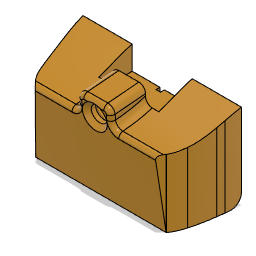
Nase+_ohne_Cam (Autodesk Fusion 360 design; units mm, degrees)
Autodesk Fusion 360 part; units mm, degrees
sketch "Skizze1" plane through (0, 0, 0) normal (1, 0, 0) x (0, 0, -1)
  line L0 (-230.1322, -57.5923) -> (-230.1322, 8.8027)
  spline S0 degree 3 poles (-230.1322, -57.5923) (-230.1323, -58.3551) (-230.2195, -59.1172) (-230.681, -61.096) (-231.1997, -62.2622) (-232.679, -64.3902) (-233.6453, -65.3172) (-235.732, -66.6453) (-236.7991, -67.0899) (-238.6452, -67.5093) (-239.3882, -67.5923) (-240.1323, -67.5923) knots -3.547857 -3.547857 -3.547857 -3.547857 -3.317948 -3.317948 -2.938178 -2.938178 -2.539541 -2.539541 -2.193953 -2.193953 -1.968953 -1.968953 -1.968953 -1.968953
  line L1 (-285.1866, -67.5923) -> (-240.1323, -67.5923)
  line L2 (-285.1866, -67.5923) -> (-291.9232, 9.4077)
  line L3 (-291.9232, 9.4077) -> (-255.1322, 12.6265)
  line L4 (-255.1322, 12.6265) -> (-255.1322, -10.5402)
  line L5 (-255.1322, -10.5402) -> (-230.1322, -10.5402)
  line L6 (-235.8283, -10.5402) -> (-205.3183, -10.5402)
  dimension "d33" = 95
  dimension "d34" = 77
  dimension "d35" = 25
  constraint coincident L1.start L2.start
  constraint perpendicular L2 L3
  constraint coincident L0 L5.end
  constraint perpendicular L0 L5
  constraint vertical L4
  constraint collinear L5 L6
  measures "d33" angle of L1 L2
  measures "d34" vertical distance of L1.start L2.end
  measures "d35" distance of L4.end L5.end
extrude "Extrusion1" add sketch "Skizze1" along normal blind 75
sketch "Skizze2" plane through (75, 0, 0) normal (1, 0, 0) x (0, 0, -1)
  line L0 (-285.1866, -67.5923) -> (-240.1323, -67.5923)
  spline S0 degree 3 poles (-240.1323, -67.5923) (-239.3882, -67.5923) (-238.6452, -67.5093) (-236.7991, -67.0899) (-235.732, -66.6453) (-233.6453, -65.3172) (-232.679, -64.3902) (-231.1997, -62.2622) (-230.681, -61.096) (-230.2195, -59.1172) (-230.1323, -58.3551) (-230.1322, -57.5923) knots 1.968953 1.968953 1.968953 1.968953 2.193953 2.193953 2.539541 2.539541 2.938178 2.938178 3.317948 3.317948 3.547857 3.547857 3.547857 3.547857
  line L1 (-230.1322, -57.5923) -> (-230.1322, -10.5402)
  line L2 (-230.1322, -10.5402) -> (-255.1322, -10.5402)
  line L3 (-255.1322, -10.5402) -> (-255.1322, 12.6265)
  line L4 (-255.1322, 12.6265) -> (-291.9232, 9.4077)
  line L5 (-291.9232, 9.4077) -> (-285.1866, -67.5923)
  spline S1 degree 3 poles (-187.9213, 18.0909) (-189.9069, 17.703) (-192.5076, 17.1904) (-206.5822, 14.3288) (-218.6816, 11.6654) (-230.1322, 8.8027) knots 0.018488 0.018488 0.018488 0.018488 0.043361 0.043361 0.124927 0.124927 0.124927 0.124927
  line L6 (-230.1322, -57.5923) -> (-230.1322, 8.8027)
  spline S2 degree 5 poles (-230.1322, 8.8027) (-230.3467, 8.7493) (-230.8612, 8.6535) (-231.8902, 8.5423) (-233.7284, 8.4713) (-236.5456, 8.5712) (-239.5754, 8.9196) (-242.5379, 9.5452) (-245.2629, 10.4061) (-247.7572, 11.3549) (-250.1266, 12.1944) (-252.0422, 12.6146) (-253.5513, 12.7135) (-254.5984, 12.6732) (-255.1322, 12.6265) knots 0 0 0 0 0 0 0.1 0.2 0.3 0.4 0.5 0.6 0.7 0.8 0.9 1 1 1 1 1 1
  line L7 (-252.49, 12.8576) -> (-257.7745, 12.3953)
  line L8 (-229.0052, 9.0833) -> (-231.2593, 8.5221)
  point P0 (-242.1322, 9.5151)
  dimension "d38" = 12
  constraint coincident S1.end L6.end
  constraint coincident L3.end L4.start
  constraint midpoint L3.end L7
  constraint collinear L4 L7
  constraint midpoint S1.end L8
  constraint coincident S1 L8.start
  measures "d38" distance of S1.end P0
extrude "Extrusion2" add sketch "Skizze2" against normal up to surface (75 mm away) contours L2 L3 L6 S2
sketch "Skizze3" plane through (0, -67.5923, 0) normal (0, -1, 0) x (1, 0, 0)
  line L0 (0, 285.1866) -> (0, 240.1322)
  line L1 (0, 240.1322) -> (75, 240.1322)
  line L2 (75, 240.1322) -> (75, 285.1866)
  line L3 (75, 285.1866) -> (0, 285.1866)
  line L4 (71.2216, 230.1322) -> (71.2222, 230.1322)
  spline S0 degree 3 poles (71.2216, 230.1322) (71.2216, 230.1323) (71.2145, 230.2195) (71.1764, 230.681) (71.1335, 231.1997) (71.0064, 232.679) (70.9214, 233.6453) (70.7281, 235.732) (70.6257, 236.7991) (70.4399, 238.6452) (70.3629, 239.3882) (70.2836, 240.1322) knots -3.547857 -3.547857 -3.547857 -3.547857 -3.317948 -3.317948 -2.938178 -2.938178 -2.539541 -2.539541 -2.193953 -2.193953 -1.968953 -1.968953 -1.968953 -1.968953
  spline S1 degree 3 poles (58.6159, 285.1866) (58.8386, 284.9235) (59.0508, 284.6534) (60.7169, 282.3992) (61.8905, 279.913) (64.5784, 273.0784) (65.9199, 267.6926) (68.3735, 255.7288) (69.468, 247.7755) (70.2836, 240.1322) knots -5.23881 -5.23881 -5.23881 -5.23881 -5.137479 -5.137479 -4.40162 -4.40162 -2.938078 -2.938078 -0.734509 -0.734509 -0.734509 -0.734509
  spline S2 degree 3 poles (58.6159, 285.1866) (58.6607, 285.1336) (58.7036, 285.082) (58.7446, 285.032) knots 2.347668 2.347668 2.347668 2.347668 2.463327 2.463327 2.463327 2.463327
  spline S3 degree 3 poles (58.7446, 285.032) (58.7446, 285.032) (58.7446, 285.032) (58.7446, 285.032) (58.7446, 285.032) (58.7447, 285.032) (58.7447, 285.032) (58.7447, 285.032) (58.745, 285.0315) (58.8339, 284.9233) (59.213, 284.4459) (59.9753, 283.3578) (60.5948, 282.3767) (61.7598, 280.0779) (62.2623, 278.9578) (63.1942, 276.6031) (63.622, 275.4007) (64.029, 274.1408) knots 0 0 0 0 0.000009 0.000009 0.000026 0.000026 0.000061 0.000061 0.00019 0.00019 0.049058 0.049058 0.12323 0.12323 0.177862 0.177862 0.227465 0.227465 0.227465 0.227465
  spline S4 degree 3 poles (64.029, 274.1408) (64.0291, 274.1406) (64.0291, 274.1405) (64.0294, 274.1398) (64.0297, 274.1389) (64.0383, 274.112) (64.0457, 274.0893) (66.2561, 267.2218) (68.1228, 257.9178) (71.2453, 232.8274) (72.1727, 218.7406) (72.8111, 200.9991) (72.9234, 196.5955) (73.004, 189.7858) (73, 187.2672) (73, 184.7764) knots 0 0 0 0 0.000068 0.000068 0.000117 0.000117 0.000383 0.000383 0.080564 0.080564 0.168272 0.168272 0.196731 0.196731 0.213685 0.213685 0.213685 0.213685
  line L5 (73, 184.7764) -> (73, 158.8712)
  line L6 (73, 133.8045) -> (73, 158.8712)
  line L7 (73, 133.8045) -> (73, 133.8187)
  line L8 (73, 184.5854) -> (73, 133.8187)
  line L9 (73, 184.5854) -> (73, 187.9213)
  spline S5 degree 3 poles (73, 187.9213) (73, 189.9069) (72.9829, 192.5076) (72.7138, 206.5822) (72.1595, 218.6816) (71.2222, 230.1322) knots 0.018488 0.018488 0.018488 0.018488 0.043361 0.043361 0.124927 0.124927 0.124927 0.124927
  spline S6 degree 3 poles (58.6159, 285.1866) (58.8386, 284.9235) (59.0508, 284.6534) (60.7169, 282.3992) (61.8905, 279.913) (64.5784, 273.0784) (65.9199, 267.6926) (68.3735, 255.7288) (69.468, 247.7755) (70.2836, 240.1322) knots -5.23881 -5.23881 -5.23881 -5.23881 -5.137479 -5.137479 -4.40162 -4.40162 -2.938078 -2.938078 -0.734509 -0.734509 -0.734509 -0.734509
  spline S7 degree 3 poles (71.2216, 230.1322) (71.2216, 230.1323) (71.2145, 230.2195) (71.1764, 230.681) (71.1335, 231.1997) (71.0064, 232.679) (70.9214, 233.6453) (70.7281, 235.732) (70.6257, 236.7991) (70.4399, 238.6452) (70.3629, 239.3882) (70.2836, 240.1322) knots -3.547857 -3.547857 -3.547857 -3.547857 -3.317948 -3.317948 -2.938178 -2.938178 -2.539541 -2.539541 -2.193953 -2.193953 -1.968953 -1.968953 -1.968953 -1.968953
  line L10 (58.7446, 285.032) -> (58.7446, 295.032)
  line L11 (58.7446, 295.032) -> (88.7446, 295.032)
  line L12 (88.7446, 295.032) -> (88.7446, 187.9213)
  line L13 (88.7446, 187.9213) -> (73, 187.9213)
  spline S8 degree 5 poles (58.7446, 285.032) (58.381, 285.4655) (57.6443, 286.3248) (56.5113, 287.5913) (54.9512, 289.2391) (52.9392, 291.2378) (51.2882, 292.7837) (50.0263, 293.9059) (49.1738, 294.6353) (48.7446, 294.9954) knots 0 0 0 0 0 0 0.2 0.4 0.6 0.8 1 1 1 1 1 1
  line L14 (59.614, 283.996) -> (57.8752, 286.0681)
  line L15 (49.7706, 294.1345) -> (47.7186, 295.8563)
  line L16 (48.7446, 294.9954) -> (58.7446, 295.032)
  line L17 (70.2836, 240.1322) -> (88.7446, 240.1322)
  line L18 (71.2216, 230.1322) -> (88.7446, 230.1322)
  line L19 (71.8416, 221.7131) -> (88.7446, 221.7131)
  dimension "d57" = 30
  dimension "d58" = 10
  dimension "d59" = 130
  dimension "d60" = 140
  dimension "d61" = 10
  constraint coincident S2.end S3.start
  constraint perpendicular L3 L10
  constraint perpendicular L10 L11
  constraint perpendicular L11 L12
  constraint coincident L9.end S5.start
  constraint perpendicular L12 L13
  constraint midpoint S2.end L14
  constraint midpoint S8.end L15
  constraint coincident S0.end S1.end
  constraint coincident L12 L17.end
  constraint perpendicular L12 L17
  constraint coincident L4.start S0.start
  constraint coincident L12 L18.end
  constraint perpendicular L12 L18
  constraint coincident S4 L19.start
  constraint coincident L12 L19.end
  constraint perpendicular L12 L19
  measures "d57" distance of L10.end L11.end
  measures "d58" distance of S2.end L11
  measures "d59" angle of L3 L14
  measures "d60" angle of L3 L15
  measures "d61" distance of L10.end S8.end
extrude "Extrusion4" cut sketch "Skizze3" against normal blind 90 contours L3 L10 S8 L16 | L1 L2 L3 S1 S4 S6 L10 L17 | L1 S4 L12 L17 L18 | L2 L3 L10 L11 L12 L17 | S4 L12 L18 L19
ref_plane "Arbeitsebene1" through (75, -27.3056, 261.0277) normal (-1, 0, 0) x (0, 0, 1)
sketch "Skizze4" plane through (75, -27.3056, 261.0277) normal (-1, 0, 0) x (0, 0, -1)
  spline S0 degree 3 poles (73.1065, -45.3966) (71.1208, -45.0087) (68.5202, -44.496) (54.4456, -41.6344) (42.3461, -38.9711) (30.8955, -36.1084) knots 0.018488 0.018488 0.018488 0.018488 0.043361 0.043361 0.124927 0.124927 0.124927 0.124927
  spline S1 degree 5 poles (30.8955, -36.1084) (29.6072, -35.7632) (27.0506, -35.0334) (23.275, -33.8203) (18.3502, -31.9995) (12.3257, -29.5658) (6.3697, -27.1974) (0.4217, -25.103) (-5.5648, -23.4248) (-11.607, -22.1682) (-17.7015, -21.2505) (-22.6089, -20.6952) (-26.3009, -20.3325) (-28.7663, -20.1079) (-30, -20) knots 0 0 0 0 0 0 0.1 0.2 0.3 0.4 0.5 0.6 0.7 0.8 0.9 1 1 1 1 1 1
  line L0 (0, 0) -> (41.8559, 0) construction
  line L1 (37.427, -37.8585) -> (24.3639, -34.3582)
  line L2 (-23.4407, -20.5739) -> (-36.5593, -19.4261)
  line L3 (-24.1589, 40.2867) -> (-30.8955, -36.7133)
  line L4 (-10.9779, -38.4559) -> (5.8955, -39.9321)
  line L5 (-24.0047, -37.3162) -> (-10.9779, -38.4559)
  line L6 (-30.8955, -36.7133) -> (-24.1589, -37.3027)
  line L7 (-30, -20) -> (-30.8955, -36.7133)
  line L8 (-30.8955, -36.7133) -> (-30.8955, -46.7133)
  line L9 (-30.8955, -46.7133) -> (30.8955, -46.7133)
  line L10 (30.8955, -46.7133) -> (30.8955, -36.1084)
  point P0 (30.8955, -36.1084)
  point P1 (-0.2494, -25)
  dimension "d65" = 20
  dimension "d66" = 25
  dimension "d67" = 15
  dimension "d68" = 5
  dimension "d69" = 10
  constraint coincident P0 S0.end
  constraint coincident L0.start origin
  constraint horizontal L0
  constraint midpoint P0 L1
  constraint midpoint S1.end L2
  constraint coincident L3.end L6.start
  constraint horizontal L9
  constraint vertical L10
  constraint vertical L8
  measures "d65" distance of L0.start S1.end
  measures "d66" vertical distance of L0.start P1
  measures "d67" angle of L0 L1
  measures "d68" angle of L0 L2
  measures "d69" distance of L3.end L8.end
extrude "Extrusion5" cut sketch "Skizze4" along normal blind 60 contours S1 L3 L8 L9 L10
sketch "Skizze5" plane through (0, 0, 230.1322) normal (0, 0, -1) x (-1, 0, 0)
  line L0 (-71.2266, 8.8027) -> (-71.2266, -57.5923)
  line L1 (-71.2266, -57.5923) -> (0, -57.5923)
  line L2 (0, -57.5923) -> (0, 8.8027)
  line L3 (0, 8.8027) -> (-15, 8.8027)
  line L4 (-15, 8.8027) -> (-71.2266, 8.8027)
  line L5 (-27, 8.8027) -> (-27, -12.3928)
  line L6 (-27, -12.3928) -> (-2, -12.3928)
  line L7 (-27, -12.3928) -> (0, -12.3928)
  line L8 (0, -12.3928) -> (0, 27.6072)
  line L9 (0, 27.6072) -> (-27, 27.6072)
  line L10 (-27, 27.6072) -> (-27, -12.3928)
  dimension "d72" = 40
  constraint horizontal L7
  constraint vertical L8
  constraint horizontal L9
  constraint vertical L10
  constraint coincident L5.end L6.start
  constraint coincident origin L8
  measures "d72" distance of L7.end L8.end
extrude "Extrusion6" cut sketch "Skizze5" against normal blind 30 contours L3 L4 L8 L9 L10 | L2 L3 L4 L5 L6 L7 L8 L10
fillet "Abrundung1" radius 6 2 edges at (15, -5.4791, 275.1636) (15, 10.7984, 276.0277)
sketch "Skizze6" plane through (0, 0, 0) normal (-1, 0, 0) x (0, 0, 1)
  line L0 (260.1322, -12.3928) -> (230.1322, -12.3928)
  line L1 (230.1322, -12.3928) -> (230.1322, -57.5923)
  spline S0 degree 3 poles (230.1322, -57.5923) (230.1323, -58.3551) (230.2195, -59.1172) (230.681, -61.096) (231.1997, -62.2622) (232.679, -64.3902) (233.6453, -65.3172) (235.732, -66.6453) (236.7991, -67.0899) (238.6452, -67.5093) (239.3882, -67.5923) (240.1323, -67.5923) knots -3.547857 -3.547857 -3.547857 -3.547857 -3.317948 -3.317948 -2.938178 -2.938178 -2.539541 -2.539541 -2.193953 -2.193953 -1.968953 -1.968953 -1.968953 -1.968953
  line L2 (240.1323, -67.5923) -> (285.1866, -67.5923)
  line L3 (285.1866, -67.5923) -> (291.9232, 9.4077)
  line L4 (291.9232, 9.4077) -> (260.1322, 12.189)
  line L5 (260.1322, 12.189) -> (260.1322, -12.3928)
  line L6 (230.1322, -12.3928) -> (233.6322, -12.3928)
  line L7 (233.6322, -12.3928) -> (233.6322, -67.5923)
  line L8 (233.6322, -67.5923) -> (230.1322, -67.5923)
  line L9 (230.1322, -67.5923) -> (230.1322, -12.3928)
  dimension "d77" = 3.5
  constraint horizontal L6
  constraint vertical L7
  constraint horizontal L8
  constraint vertical L9
  constraint coincident L0.end L1.start
  constraint collinear L2 L8
  measures "d77" distance of L7.end L8.end
extrude "Extrusion7" cut sketch "Skizze6" against normal blind 2 contours L0 L1 S0 L6 L7 L9
sketch "Skizze7" plane through (0, 0, 0) normal (-1, 0, 0) x (0, 0, 1)
  line L0 (233.6322, -12.3928) -> (233.6322, -65.1916)
  spline S0 degree 3 poles (233.6322, -65.1916) (233.9884, -65.4962) (234.3661, -65.776) (235.732, -66.6453) (236.7991, -67.0899) (238.6452, -67.5093) (239.3882, -67.5923) (240.1323, -67.5923) knots -2.681083 -2.681083 -2.681083 -2.681083 -2.539541 -2.539541 -2.193953 -2.193953 -1.968953 -1.968953 -1.968953 -1.968953
  line L1 (240.1323, -67.5923) -> (285.1866, -67.5923)
  line L2 (285.1866, -67.5923) -> (291.9232, 9.4077)
  line L3 (291.9232, 9.4077) -> (260.1322, 12.189)
  line L4 (260.1322, 12.189) -> (260.1322, -12.3928)
  line L5 (260.1322, -12.3928) -> (233.6322, -12.3928)
  line L6 (286.6818, 6.8665) -> (260.1322, 9.1893)
  line L7 (260.1322, 9.1893) -> (260.1322, -12.3928)
  line L8 (286.6818, 6.8665) -> (284.8079, -14.5516)
  line L9 (284.8079, -14.5516) -> (260.1322, -12.3928)
  dimension "d80" = 21.5
  dimension "d81" = 5
  constraint perpendicular L2 L6
  constraint coincident L5 L4.end
  constraint perpendicular L5 L7
  constraint perpendicular L6 L8
  constraint parallel L6 L9
  constraint coincident L4.end L5.start
  measures "d80" distance of L6.start L8.end
  measures "d81" distance of L2 L8
extrude "Extrusion8" cut sketch "Skizze7" against normal blind 10 contours L4 L6 L7 L8 L9
sketch "Skizze8" plane through (0, -24.8387, 283.9079) normal (0, 0.087156, -0.996195) x (-1, 0, 0)
  line L0 (0, 10.3264) -> (0, 31.8264)
  line L1 (0, 31.8264) -> (-10, 31.8264)
  line L2 (-10, 31.8264) -> (-10, 10.3264)
  line L3 (-10, 10.3264) -> (0, 10.3264)
  circle A0 centre (0, 21.0764) radius 7.15
  dimension "d84" = 14.3
  constraint midpoint L0 A0.centre
  measures "d84" diameter of A0
extrude "Extrusion9" cut sketch "Skizze8" against normal blind 8 contours L0 A0 picked at (-3.6851, 22.9043)
extrude "Extrusion10" add 1 faces at (4.3674, 5.436, 286.5566) along direction (0, 0.087156, -0.996195) blind 5
fillet "Abrundung2" radius 2 1 edges at (7.15, -3.4068, 280.7639)
chamfer "Fase1" distance 4 angle 45 1 edges at (7.15, -4.2783, 290.7258)
sketch "Skizze9" plane through (10, 0, 0) normal (-1, 0, 0) x (0, 0, 1)
  line L0 (279.827, -14.1159) -> (281.7008, 7.3023)
  line L1 (281.7008, 7.3023) -> (260.1322, 9.1893)
  line L2 (260.1322, 9.1893) -> (260.1322, -12.3928)
  line L3 (260.1322, -12.3928) -> (279.827, -14.1159)
  spline S0 degree 3 poles (290.4653, -7.2561) (287.9411, -7.0319) (285.4058, -6.787) (280.315, -6.2169) (277.752, -5.8899) (275.1636, -5.4791) (272.5886, -5.0704) (269.9916, -4.5763) (264.9559, -3.3915) (262.5176, -2.7105) (260.1322, -1.9463) knots -6.169471 -6.169471 -6.169471 -6.169471 -5.419728 -5.419728 -4.669986 -4.669986 -4.669986 -3.924136 -3.924136 -3.216523 -3.216523 -3.216523 -3.216523
  spline S1 degree 3 poles (290.3061, -9.049) (287.7725, -8.8241) (285.2235, -8.5779) (282.6601, -8.2908) (280.0962, -8.0036) (277.5055, -7.6733) (274.8814, -7.2568) (272.2697, -6.8423) (269.6295, -6.3403) (266.9953, -5.7205) (264.4952, -5.1323) (262.0119, -4.4386) (259.5831, -3.6605) knots -6.169471 -6.169471 -6.169471 -6.169471 -5.419728 -5.419728 -5.419728 -4.669986 -4.669986 -4.669986 -3.924136 -3.924136 -3.924136 -3.216523 -3.216523 -3.216523 -3.216523
  dimension "d92" = -1.8
extrude "Extrusion11" cut sketch "Skizze9" against normal up to surface (17 mm away) contours L0 L2 L3 S1
chamfer "Fase2" distance 5 angle 45 2 edges at (27, -6.3766, 269.9937) (27, -11.0686, 280.0936)
fillet "Abrundung3" radius 4 5 edges at (4.5, 9.4077, 291.9232) (13.2426, 7.657, 291.77) (15, 1.0758, 291.1943) (16.7555, -5.5035, 290.6186) (37.3505, -7.2561, 290.4653)
mirror "Spiegeln1" about plane through (0, -10.9653, 285.1217) normal (-1, 0, 0) of bodies 1 merged
